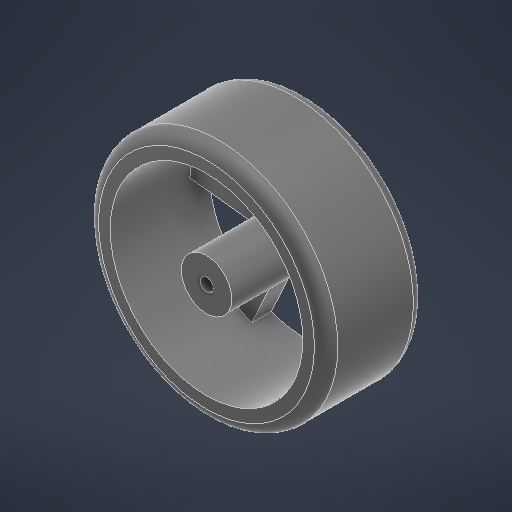
# Autodesk Inventor part: OGWheel
Saved by Autodesk Inventor 2027 (Build 310192060, 192F)
## iProperties
Created: 2026-07-12
Part Number: OGWheel
Material: ABS Plastic
Document SubType Name: Modeling
Designer: machnach0
Density: 1.06 g/cm^3
Appearance: Smooth - Black
Author: machnach0
Autodesk Inventor part; units mm, degrees
ref_plane "YZ Plane" through (0, 0, 0) normal (1, 0, 0) x (0, 1, 0)
ref_plane "XZ Plane" through (0, 0, 0) normal (0, 1, 0) x (-1, 0, 0)
ref_plane "XY Plane" through (0, 0, 0) normal (0, 0, 1) x (1, 0, 0)
sketch "Sketch1" plane through (0, 0, 0) normal (0, 0, 1) x (1, 0, 0)
  circle A0 centre (0, 0) radius 1.778
  circle A1 centre (0, 0) radius 32.512
  circle A2 centre (0, 0) radius 26.162
  circle A3 centre (0, 0) radius 6.858
  line L0 (-3.048, 6.1434) -> (-6.8485, 25.2497)
  line L1 (3.048, 6.1434) -> (6.8485, 25.2497)
  arc A4 (6.8485, 25.2497) -> (-6.8485, 25.2497) centre (0, 0) ccw construction
  line L2 (-6.7846, -1.0004) -> (-26.1302, 1.2893)
  circle A5 centre (0, 0) radius 26.162
  line L3 (-4.9009, 4.7972) -> (-21.8976, 14.3159)
  circle A6 centre (0, 0) radius 6.858
  line L4 (-1.1451, -6.7617) -> (-9.3009, -24.4529)
  circle A7 centre (0, 0) radius 26.162
  line L5 (-6.0769, -3.1786) -> (-20.3819, -16.402)
  circle A8 centre (0, 0) radius 6.858
  line L6 (6.0769, -3.1786) -> (20.3819, -16.402)
  circle A9 centre (0, 0) radius 26.162
  line L7 (1.1451, -6.7617) -> (9.3009, -24.4529)
  circle A10 centre (0, 0) radius 6.858
  line L8 (4.9009, 4.7972) -> (21.8976, 14.3159)
  circle A11 centre (0, 0) radius 26.162
  line L9 (6.7846, -1.0004) -> (26.1302, 1.2893)
  circle A12 centre (0, 0) radius 6.858
  dimension "d1" = 65.024
  dimension "d2" = 3.556
  dimension "d3" = 13.716
  dimension "d4" = 6.35
  dimension "d5" = 22.5
  dimension "d7" = 3.048
  dimension "d10" = 360
  constraints: 22 point on circle, 20 end point, 13 centre point, 7 coincident, 2 horizontal alignment, 1 concentric, 51 other
  measures "d1" diameter of A1
  measures "d2" diameter of A0
  measures "d3" diameter of A3
  measures "d4" radial gap between concentric circles of A1 A2
  measures "d5" angle of L1 L0
  measures "d7" horizontal distance of point (0, 0) L0.start
extrude "Extrusion1" add sketch "Sketch1" along normal blind 26.924 contours A1 | A3
extrude "Extrusion2" add sketch "Sketch1" along normal blind 21.59 contours A0
extrude "Extrusion3" add sketch "Sketch1" along normal blind 5.334 contours L9 A3 L8 A2 | A2 L7 A3 L6 | L1 A3 L0 A2 | A2 L5 A3 L4 | L3 A3 L2 A2
fillet "Fillet1" radius 3.175 2 edges at (-32.512, 0, 26.924) (-32.512, 0, 0)
body "Solid1"
